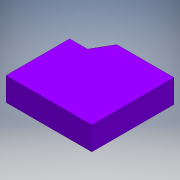
# Autodesk Inventor part: Cam_SD_base
Saved by Autodesk Inventor 2018 (Build 220112000, 112)
## iProperties
Created: 2018-05-25
Part Number: Cam_SD_base
Material: Generic
Document SubType Name: Modeling
Designer: Suchanek
Density: 1 g/cm^3
Appearance: Default
Author: Suchanek
Autodesk Inventor part; units mm, degrees
ref_plane "YZ Plane" through (0, 0, 0) normal (1, 0, 0) x (0, 1, 0)
ref_plane "XZ Plane" through (0, 0, 0) normal (0, 1, 0) x (-1, 0, 0)
ref_plane "XY Plane" through (0, 0, 0) normal (0, 0, 1) x (1, 0, 0)
sketch "Sketch1" plane through (0, 0, 0) normal (0, 0, 1) x (1, 0, 0)
  line L0 (0, 0) -> (-24, 0)
  line L1 (-24, 0) -> (-24, 23)
  line L2 (-24, 23) -> (0, 23)
  line L3 (0, 23) -> (0, 0)
  line L4 (-24, 17.8038) -> (-19, 17.8038)
  line L5 (-19, 17.8038) -> (-16, 23)
  dimension "d0" = 23
  dimension "d1" = 24
  dimension "d2" = 120
  dimension "d3" = 5
  dimension "d4" = 6
  constraints: 12 end point, 2 horizontal, 2 parallel, 2 point on line, 1 perpendicular
  measures "d0" distance of L2.end L0.start
  measures "d1" distance of L1.end L2.end
  measures "d2" angle of L5 L4
  measures "d3" distance of L4.start L4.end
  measures "d4" distance of L4.end L5.end
extrude "Extrusion1" add sketch "Sketch1" along normal blind 6.5 contours L0 L1 L4 L5 L2 L3
body "Solid1"
